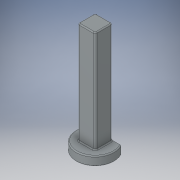
# Autodesk Inventor part: Axle 2
Saved by Autodesk Inventor 2019 (Build 230136000, 136)
## iProperties
Company: Unknown
Created: 2018-11-05
Part Number: Axle 2
Material: Generic
Description: Unknown
Document SubType Name: Modeling
Designer: Varga Daniel
Density: 1 g/cm^3
Appearance: Default
Sending System: DEX
Preprocessor: ST-DEVELOPER v16.7
Title: Axeis 2
Author: Unknown
Autodesk Inventor part; units mm, degrees
ref_plane "YZ Plane" through (0, 0, 0) normal (1, 0, 0) x (0, 1, 0)
ref_plane "XZ Plane" through (0, 0, 0) normal (0, 1, 0) x (-1, 0, 0)
ref_plane "XY Plane" through (0, 0, 0) normal (0, 0, 1) x (1, 0, 0)
feature "Base1" [suppressed]
sketch "Sketch1" plane through (0, 0, 0) normal (0, 1, 0) x (-1, 0, 0)
  line L0 (-1.325, -1.725) -> (1.325, -1.725)
  line L1 (1.725, -1.325) -> (1.725, 1.325)
  line L2 (1.325, 1.725) -> (-1.325, 1.725)
  line L3 (-1.725, 1.325) -> (-1.725, -1.325)
  line L4 (-1.725, -1.725) -> (1.725, 1.725) construction
  line L5 (1.725, -1.725) -> (-1.725, 1.725) construction
  arc A0 (-1.725, -1.325) -> (-1.325, -1.725) centre (-1.325, -1.325) ccw
  arc A1 (1.325, -1.725) -> (1.725, -1.325) centre (1.325, -1.325) ccw
  arc A2 (1.725, 1.325) -> (1.325, 1.725) centre (1.325, 1.325) ccw
  arc A3 (-1.325, 1.725) -> (-1.725, 1.325) centre (-1.325, 1.325) ccw
  point P0 (0, 0)
  dimension "d0" = 3.45
  dimension "d1" = 3.45
  dimension "d2" = 0.4
  constraints: 12 end point, 8 point on circle, 8 point on line, 8 tangent, 4 centre point, 3 equal radius, 2 midpoint, 2 parallel, 1 horizontal, 1 perpendicular
  measures "d0" distance of L4.end L5.end
  measures "d1" distance between parallel lines of L2 L0
  measures "d2" radius of A0
extrude "Extrusion1" add sketch "Sketch1" along normal blind 20
sketch "Sketch2" plane through (0, 0, 0) normal (0, -1, 0) x (1, 0, 0)
  circle A0 centre (0, 0) radius 3.75
  dimension "d5" = 7.5
  constraints: 1 centre point, 1 coincident
  measures "d5" diameter of A0
extrude "Extrusion2" add sketch "Sketch2" along normal blind 1.8
fillet "Fillet1" radius 0.2 18 edges at (-1.6078, 20, 1.6078) (0, 20, 1.725) (1.6078, 20, 1.6078) (1.725, 20, 0) (1.6078, 20, -1.6078) (0, 20, -1.725) (-1.6078, 20, -1.6078) (-1.725, 20, 0) (-1.6078, 0, 1.6078) (0, 0, 1.725) (1.6078, 0, 1.6078) (1.725, 0, 0) (1.6078, 0, -1.6078) (0, 0, -1.725) (-1.6078, 0, -1.6078) (-1.725, 0, 0) (-3.75, 0, 0) (-3.75, -1.8, 0)
sketch "Sketch3" plane through (1.325, 0.2, -1.725) normal (0, 0, -1) x (-1, 0, 0)
  line L0 (-6.9132, 22.2814) -> (9.6006, 22.2814)
  line L1 (9.6006, 22.2814) -> (9.6006, -8.1567)
  line L2 (9.6006, -8.1567) -> (-6.9132, -8.1567)
  line L3 (-6.9132, -8.1567) -> (-6.9132, 22.2814)
  point P0 (1.325, -0.2)
  constraints: 8 end point, 2 parallel, 1 horizontal, 1 perpendicular
extrude "Extrusion3" cut sketch "Sketch3" along normal through all
equation "\"d1\" = d0"
body "Solid1"
